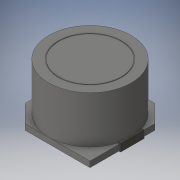
# Autodesk Inventor part: SRR7045-151M
Saved by Autodesk Inventor 2016 (Build 200138000, 138)
## iProperties
Created: 2016-08-10
Part Number: SRR7045-151M
Material: Generic
Document SubType Name: Modeling
Designer: jfixelle
Density: 1 g/cm^3
Appearance: Gray
Author: jfixelle
Autodesk Inventor part; units mm, degrees
ref_plane "YZ Plane" through (0, 0, 0) normal (1, 0, 0) x (0, 1, 0)
ref_plane "XZ Plane" through (0, 0, 0) normal (0, 1, 0) x (-1, 0, 0)
ref_plane "XY Plane" through (0, 0, 0) normal (0, 0, 1) x (1, 0, 0)
sketch "Sketch1" plane through (0, 0, 0) normal (0, 1, 0) x (-1, 0, 0)
  line L0 (3.5, 3.5) -> (-3.5, 3.5)
  line L1 (-3.5, 3.5) -> (-3.5, -3.5)
  line L2 (-3.5, -3.5) -> (3.5, -3.5)
  line L3 (3.5, -3.5) -> (3.5, 3.5)
  line L4 (3.5, 2) -> (2, 3.5)
  line L5 (-2, -3.5) -> (-3.5, -2)
  point P0 (0, 0)
  dimension "d0" = 7
  dimension "d1" = 7
  dimension "d2" = 3.5
  dimension "d3" = 3.5
  dimension "d4" = 45
  dimension "d5" = 45
  dimension "d6" = 5.5
  dimension "d7" = 5.5
  constraints: 12 end point, 4 point on line, 2 parallel, 1 horizontal, 1 perpendicular
  measures "d0" distance of L2.end L0.start
  measures "d1" distance of L1.end L2.end
  measures "d2" distance from line of point (0, 0) L3
  measures "d3" distance from line of point (0, 0) L2
  measures "d4" angle of L2 L5
  measures "d5" angle of L3 L4
  measures "d6" distance from line of L3 L5.start
  measures "d7" distance from line of L4.end L1
extrude "Extrusion1" add sketch "Sketch1" along normal blind 0.5 contours L4 L3 L2 L5 L1 L0
sketch "Sketch2" plane through (0, 0.5, 0) normal (0, 1, 0) x (1, 0, 0)
  circle A0 centre (0, 0) radius 3.5
  dimension "d10" = 7
  constraints: 1 centre point, 1 coincident
  measures "d10" diameter of A0
extrude "Extrusion2" add sketch "Sketch2" along normal blind 4
sketch "Sketch3" plane through (0, 4.5, 0) normal (0, 1, 0) x (1, 0, 0)
  circle A0 centre (0, 0) radius 2.6934
  circle A1 centre (0, 0) radius 2.6335
  constraints: 2 centre point, 2 coincident
extrude "Extrusion3" cut sketch "Sketch3" against normal blind 0.05
sketch "Sketch4" plane through (0, 0, 0) normal (0, -1, 0) x (1, 0, 0)
  line L0 (3.5, 3.5) -> (3.5, 0) projected
  line L1 (3.5, 1) -> (2, 1)
  line L2 (2, 1) -> (2, -1)
  line L3 (2, -1) -> (3.5, -1)
  line L4 (3.5, -1) -> (3.5, 1)
  line L5 (-2, 3.5) -> (3.5, 3.5) projected
  point P0 (0, 0)
  dimension "d15" = 1.5
  dimension "d16" = 2
  dimension "d17" = 2.5
  constraints: 8 end point, 2 parallel, 1 horizontal, 1 perpendicular, 1 point on line
  measures "d15" distance of L2.end L3.end
  measures "d16" distance of L3.end L1.start
  measures "d17" distance between parallel lines of L5 L1
extrude "Extrusion4" cut sketch "Sketch4" against normal blind 0.6
sketch "Sketch5" plane through (0, 0.6, 0) normal (0, -1, 0) x (1, 0, 0)
  line L0 (2, -1) -> (2, 1) projected
  line L1 (3.6, 1) -> (2, 1)
  line L2 (2, 1) -> (2, -1)
  line L3 (2, -1) -> (3.6, -1)
  line L4 (3.6, -1) -> (3.6, 1)
  point P0 (0, 0)
  dimension "d20" = 2
  dimension "d21" = 1.6
  constraints: 8 end point, 2 parallel, 1 horizontal, 1 perpendicular
  measures "d20" distance of L3.end L1.start
  measures "d21" distance between parallel lines of L0 L4
extrude "Extrusion5" add sketch "Sketch5" along normal blind 0.65
mirror "Mirror1" about plane through (0, 0, 0) normal (1, 0, 0) of "Extrusion4"
mirror "Mirror2" about plane through (0, 0, 0) normal (1, 0, 0) of "Extrusion5"
body "Solid1"
